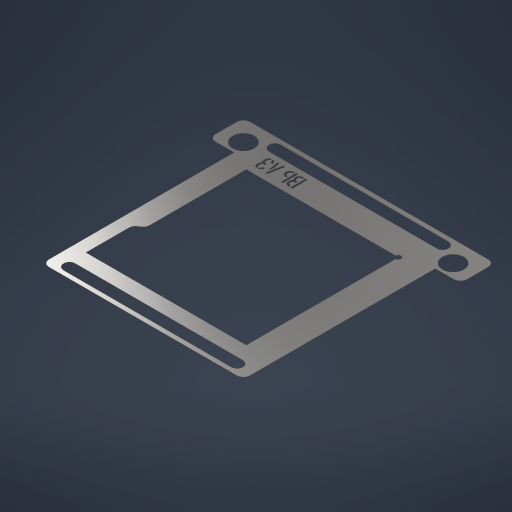
# Autodesk Inventor part: Baseplate Film Stencil - V1
Saved by Autodesk Inventor 2024 (Build 280153000, 153)
## iProperties
Created: 2022-06-23
Part Number: Baseplate Film Stencil - V1
Material: Stainless Steel
Document SubType Name: Modeling
Designer: Caleb
Density: 8 g/cm^3
Appearance: Semi-Polished
Author: Caleb
Autodesk Inventor part; units mm, degrees
ref_plane "YZ Plane" through (0, 0, 0) normal (1, 0, 0) x (0, 1, 0)
ref_plane "XZ Plane" through (0, 0, 0) normal (0, 1, 0) x (-1, 0, 0)
ref_plane "XY Plane" through (0, 0, 0) normal (0, 0, 1) x (1, 0, 0)
sketch "Sketch1" plane through (0, 0, 0) normal (0, 1, 0) x (-1, 0, 0)
  line L0 (-38.1, -34.29) -> (38.1, -34.29)
  line L1 (38.1, -34.29) -> (38.1, 34.29)
  line L2 (38.1, 34.29) -> (-38.1, 34.29)
  line L3 (-38.1, 34.29) -> (-38.1, -34.29)
  line L4 (-38.1, -34.29) -> (38.1, 34.29) construction
  line L5 (38.1, -34.29) -> (-38.1, 34.29) construction
  point P0 (0, 0)
  dimension "d0" = 76.2
  dimension "d1" = 68.58
  constraints: 12 end point, 2 midpoint, 2 parallel, 1 horizontal, 1 perpendicular
  measures "d0" distance of L2.end L1.end
  measures "d1" distance of L1.end L0.end
extrude "Extrusion1" add sketch "Sketch1" along normal blind 0.0508
sketch "Sketch2" plane through (0, 0.0508, 0) normal (0, 1, 0) x (1, 0, 0)
  line L0 (-38.1, -34.29) -> (38.1, -34.29) projected
  line L1 (-46.3971, 0) -> (43.7494, 0)
  line L2 (-38.1, 34.29) -> (-38.1, -34.29) projected
  line L3 (38.1, -34.29) -> (38.1, 34.29) projected
  line L4 (38.1, 23.79) -> (30.48, 23.79)
  line L5 (30.48, 23.79) -> (30.48, -34.29)
  line L6 (30.48, -34.29) -> (38.1, -34.29)
  line L7 (38.1, -34.29) -> (38.1, 23.79)
  line L8 (0, -45.6355) -> (0, 71.8702)
  line L9 (46.3971, 0) -> (-43.7494, 0)
  line L10 (-38.1, -34.29) -> (-38.1, 34.29)
  line L11 (-38.1, 23.79) -> (-30.48, 23.79)
  line L12 (-30.48, 23.79) -> (-30.48, -34.29)
  line L13 (-30.48, -34.29) -> (-38.1, -34.29)
  line L14 (-38.1, -34.29) -> (-38.1, 23.79)
  line L15 (38.1, 34.29) -> (-38.1, 34.29) projected
  point P0 (0, 0)
  point P1 (38.1, -27.305)
  dimension "d14" = 7.62
  dimension "d16" = 10.5
  constraints: 24 end point, 6 symmetric about line, 3 point on line, 2 horizontal, 2 parallel, 1 perpendicular, 1 vertical
  measures "d14" distance of L5.end L6.end
  measures "d16" distance between parallel lines of L15 L4
extrude "Extrusion2" cut sketch "Sketch2" against normal through all contours L2 L1 L12 L0 | L2 L11 L12 L1 | L5 L1 L3 L0 | L5 L4 L3 L1
sketch "Sketch6" plane through (0, 0.0508, 0) normal (0, 1, 0) x (1, 0, 0)
  line L0 (38.1, 34.29) -> (-38.1, 34.29) projected
  line L1 (-38.1, 34.29) -> (-38.1, 23.79) projected
  line L2 (38.1, 23.79) -> (38.1, 34.29) projected
  point P0 (0, 0)
  point P1 (-31.75, 27.94)
  point P2 (31.75, 27.94)
  point P3 (36.1, 34.29)
  point P4 (-36.1, 34.29)
  point P5 (-38.1, 32.29)
  point P6 (-38.1, 25.29)
  point P7 (38.1, 25.29)
  point P8 (38.1, 32.29)
  point P9 (38.1, 28.79)
  dimension "d41" = 6.35
  dimension "d42" = 6.35
  dimension "d43" = 6.35
  constraints: 1 horizontal alignment, 1 point on line
  measures "d41" distance from line of L0 point (-31.75, 27.94)
  measures "d42" distance from line of L1 point (-31.75, 27.94)
  measures "d43" horizontal distance of point (38.1, 28.79) point (31.75, 27.94)
hole "Hole1" at (-31.75, 0.0508, -27.94) at (31.75, 0.0508, -27.94) direction (0, -1, 0) diameter 6.477 end through all
sketch "Sketch3" plane through (0, 0.0508, 0) normal (0, 1, 0) x (1, 0, 0)
  line L0 (25.4, -31.115) -> (-25.4, -31.115) construction
  line L1 (25.4, -29.365) -> (-25.4, -29.365)
  line L2 (-25.4, -32.865) -> (25.4, -32.865)
  arc A0 (25.4, -32.865) -> (25.4, -29.365) centre (25.4, -31.115) ccw
  arc A1 (-25.4, -29.365) -> (-25.4, -32.865) centre (-25.4, -31.115) ccw
  line L3 (25.4, 31.115) -> (-25.4, 31.115) construction
  line L4 (25.4, 32.865) -> (-25.4, 32.865)
  line L5 (-25.4, 29.365) -> (25.4, 29.365)
  arc A2 (25.4, 29.365) -> (25.4, 32.865) centre (25.4, 31.115) ccw
  arc A3 (-25.4, 32.865) -> (-25.4, 29.365) centre (-25.4, 31.115) ccw
  line L6 (38.1, 34.29) -> (-38.1, 34.29) projected
  line L7 (-38.1, -34.29) -> (38.1, -34.29) projected
  point P0 (0, 0)
  point P1 (0, -31.115)
  point P2 (0, 31.115)
  dimension "d17" = 3.5
  dimension "d18" = 3.5
  dimension "d19" = 50.8
  dimension "d20" = 50.8
  dimension "d21" = 3.175
  dimension "d22" = 3.175
  constraints: 16 end point, 8 point on circle, 8 tangent, 4 centre point, 3 parallel, 2 midpoint, 2 vertical alignment, 1 horizontal
  measures "d17" distance between parallel lines of L2 L1
  measures "d18" distance between parallel lines of L4 L5
  measures "d19" distance of L0.end L0.start
  measures "d20" distance of L3.end L3.start
  measures "d21" distance from line of L6 point (0, 31.115)
  measures "d22" distance from line of L7 point (0, -31.115)
extrude "Extrusion3" cut sketch "Sketch3" against normal through all
sketch "Sketch4" plane through (0, 0.0508, 0) normal (0, 1, 0) x (1, 0, 0)
  line L0 (-24.105, -24.825) -> (21.895, -24.825)
  line L1 (21.895, -24.825) -> (21.895, 21.175)
  line L2 (21.895, 21.175) -> (-24.105, 21.175)
  line L3 (-24.105, 21.175) -> (-24.105, -24.825)
  line L4 (38.1, 34.29) -> (-38.1, 34.29) projected
  line L5 (38.1, 23.79) -> (38.1, 34.29) projected
  circle A0 centre (21.895, 21.175) radius 0.7938
  circle A1 centre (31.75, 27.94) radius 3.2385 projected
  point P0 (0, 0)
  point P1 (21.895, 20.3813)
  point P2 (21.1012, 21.175)
  point P3 (29.845, 22.225)
  dimension "d29" = 1.5875
  dimension "d34" = 46
  dimension "d35" = 46
  dimension "d51" = 1.905
  dimension "d52" = 5.715
  dimension "d53" = 7.95
  dimension "d54" = 1.05
  constraints: 8 end point, 2 parallel, 1 centre point, 1 coincident, 1 horizontal, 1 perpendicular
  measures "d29" diameter of A0
  measures "d34" distance of L0.start L0.end
  measures "d35" distance of L2.end L0.start
  measures "d51" horizontal distance of point (29.845, 22.225) A1.centre
  measures "d52" vertical distance of point (29.845, 22.225) A1.centre
  measures "d53" distance from line of L1 point (29.845, 22.225)
  measures "d54" distance from line of L2 point (29.845, 22.225)
extrude "Extrusion4" cut sketch "Sketch4" against normal through all contours L3 L2 A0 L1 L0 | A0 L2 L1 | L1 L2 A0
sketch "Sketch5" plane through (0, 0.0508, 0) normal (0, 1, 0) x (1, 0, 0)
  line L0 (-24.105, -24.825) -> (-24.105, 21.175) projected
  line L1 (-24.105, -24.825) -> (-26.605, -24.825)
  line L2 (-26.605, -24.825) -> (-26.605, -9.825)
  line L3 (-26.605, -9.825) -> (-24.105, -9.825)
  line L4 (-24.105, -9.825) -> (-24.105, -24.825)
  point P0 (0, 0)
  point P1 (-24.105, -9.825)
  dimension "d36" = 15
  dimension "d37" = 2.5
  constraints: 8 end point, 2 parallel, 1 horizontal, 1 perpendicular
  measures "d36" distance of L1.end L2.end
  measures "d37" distance of L2.end L3.end
extrude "Extrusion5" cut sketch "Sketch5" against normal through all
fillet "Fillet2" radius 2 8 edges at (30.48, 0.0254, 34.29) (-30.48, 0.0254, 34.29) (-38.1, 0.0254, -23.79) (-38.1, 0.0254, -34.29) (38.1, 0.0254, -34.29) (38.1, 0.0254, -23.79) (-24.105, 0.0254, 9.825) (-26.605, 0.0254, 9.825)
sketch "Sketch8" plane through (0, 0, 0) normal (0, -1, 0) x (1, 0, 0)
  line L0 (-11.9362, -27.7477) -> (-25.3264, -27.7477) construction
  line L1 (-25.3264, -27.7477) -> (-25.3264, -23.0961) construction
  line L2 (-25.3264, -23.0961) -> (-11.9362, -23.0961) construction
  line L3 (-11.9362, -23.0961) -> (-11.9362, -27.7477) construction
  spline S0 degree 2 poles (-13.4121, -27.2933) (-13.6942, -27.287) (-14.0545, -26.9799) (-14.0608, -26.748) knots 0 0 0 1 2 2 2
  line L4 (-14.0608, -26.748) -> (-14.0608, -26.2717)
  spline S1 degree 2 poles (-14.0608, -26.2717) (-14.0545, -26.043) (-13.6816, -25.739) (-13.3996, -25.7327) knots 0 0 0 1 2 2 2
  line L5 (-13.3996, -25.7327) -> (-13.221, -25.7327)
  line L6 (-13.221, -25.7327) -> (-13.221, -25.2313)
  line L7 (-13.221, -25.2313) -> (-13.3996, -25.2313)
  spline S2 degree 2 poles (-13.3996, -25.2313) (-13.6816, -25.2251) (-14.0545, -24.918) (-14.0608, -24.6861) knots 0 0 0 1 2 2 2
  line L8 (-14.0608, -24.6861) -> (-14.0608, -24.2129)
  spline S3 degree 2 poles (-14.0608, -24.2129) (-14.0545, -23.9873) (-13.6816, -23.7146) (-13.3996, -23.7115) knots 0 0 0 1 2 2 2
  line L9 (-13.3996, -23.7115) -> (-13.221, -23.7115)
  line L10 (-13.221, -23.7115) -> (-13.221, -23.2226)
  line L11 (-13.221, -23.2226) -> (-13.3996, -23.2226)
  spline S4 degree 2 poles (-13.3996, -23.2226) (-13.6879, -23.2226) (-14.2457, -23.4577) (-14.6123, -23.9026) (-14.6186, -24.2191) knots 0 0 0 1 2 3 3 3
  line L12 (-14.6186, -24.2191) -> (-14.6186, -24.7174)
  spline S5 degree 2 poles (-14.6186, -24.7174) (-14.6155, -24.9462) (-14.3898, -25.341) (-14.1893, -25.482) knots 0 0 0 1 2 2 2
  spline S6 degree 2 poles (-14.1893, -25.482) (-14.3898, -25.6199) (-14.6155, -26.0116) (-14.6186, -26.2404) knots 0 0 0 1 2 2 2
  line L13 (-14.6186, -26.2404) -> (-14.6186, -26.7418)
  spline S7 degree 2 poles (-14.6186, -26.7418) (-14.6123, -27.0551) (-14.2426, -27.5001) (-13.6848, -27.7414) (-13.3996, -27.7414) knots 0 0 0 1 2 3 3 3
  line L14 (-13.3996, -27.7414) -> (-13.221, -27.7414)
  line L15 (-13.221, -27.7414) -> (-13.221, -27.2933)
  line L16 (-13.221, -27.2933) -> (-13.4121, -27.2933)
  line L17 (-12.4689, -23.2226) -> (-12.7008, -23.2226)
  line L18 (-12.7008, -23.2226) -> (-12.7008, -27.7414)
  line L19 (-12.7008, -27.7414) -> (-12.4689, -27.7414)
  spline S8 degree 2 poles (-12.4689, -27.7414) (-12.3341, -27.7414) (-12.1806, -27.6443) (-12.1806, -27.5315) knots 0 0 0 1 2 2 2
  line L20 (-12.1806, -27.5315) -> (-12.1806, -23.4357)
  spline S9 degree 2 poles (-12.1806, -23.4357) (-12.1806, -23.3166) (-12.3341, -23.2226) (-12.4689, -23.2226) knots 0 0 0 1 2 2 2
  line L21 (-15.2736, -23.2226) -> (-15.4114, -23.2226)
  spline S10 degree 2 poles (-15.4114, -23.2226) (-15.4898, -23.2258) (-15.5995, -23.3198) (-15.6026, -23.3887) knots 0 0 0 1 2 2 2
  line L22 (-15.6026, -23.3887) -> (-15.6026, -27.7414)
  line L23 (-15.6026, -27.7414) -> (-15.2736, -27.7414)
  spline S11 degree 2 poles (-15.2736, -27.7414) (-15.1952, -27.7383) (-15.0855, -27.6411) (-15.0824, -27.5691) knots 0 0 0 1 2 2 2
  line L24 (-15.0824, -27.5691) -> (-15.0824, -23.3887)
  spline S12 degree 2 poles (-15.0824, -23.3887) (-15.0855, -23.3198) (-15.1952, -23.2258) (-15.2736, -23.2226) knots 0 0 0 1 2 2 2
  line L25 (-16.1165, -25.6732) -> (-16.1165, -25.2313)
  line L26 (-16.1165, -25.2313) -> (-16.245, -25.2313)
  spline S13 degree 2 poles (-16.245, -25.2313) (-16.5176, -25.2313) (-17.0347, -25.457) (-17.3825, -25.8737) (-17.4045, -26.1683) knots 0 0 0 1 2 3 3 3
  spline S14 degree 2 poles (-17.4045, -26.1683) (-17.4139, -26.4754) (-17.4045, -26.7856) knots 0 0 0 1 1 1
  spline S15 degree 2 poles (-17.4045, -26.7856) (-17.3888, -27.0802) (-17.041, -27.5064) (-16.5176, -27.7383) (-16.245, -27.7414) knots 0 0 0 1 2 3 3 3
  line L27 (-16.245, -27.7414) -> (-16.1165, -27.7414)
  line L28 (-16.1165, -27.7414) -> (-16.1165, -27.2933)
  line L29 (-16.1165, -27.2933) -> (-16.2575, -27.2933)
  spline S16 degree 2 poles (-16.2575, -27.2933) (-16.5239, -27.287) (-16.8717, -26.9799) (-16.878, -26.748) knots 0 0 0 1 2 2 2
  spline S17 degree 2 poles (-16.878, -26.748) (-16.8905, -26.6164) (-16.8811, -26.3532) (-16.878, -26.2184) knots 0 0 0 1 2 2 2
  spline S18 degree 2 poles (-16.878, -26.2184) (-16.8717, -25.9928) (-16.5239, -25.6795) (-16.2575, -25.6732) knots 0 0 0 1 2 2 2
  line L30 (-16.2575, -25.6732) -> (-16.1165, -25.6732)
  line L31 (-18.9964, -27.6443) -> (-19.83, -23.326)
  spline S19 degree 2 poles (-19.83, -23.326) (-19.8519, -23.2508) (-19.9208, -23.2195) (-19.971, -23.2226) knots 0 0 0 1 2 2 2
  line L32 (-19.971, -23.2226) -> (-20.2561, -23.2226)
  spline S20 degree 2 poles (-20.2561, -23.2226) (-20.2875, -23.2226) (-20.3314, -23.2289) (-20.3502, -23.2414) knots 0 0 0 1 2 2 2
  line L33 (-20.3502, -23.2414) -> (-19.8362, -25.9646)
  line L34 (-19.8362, -25.9646) -> (-19.5103, -27.6568)
  spline S21 degree 2 poles (-19.5103, -27.6568) (-19.5009, -27.707) (-19.4602, -27.7383) (-19.4132, -27.7414) knots 0 0 0 1 2 2 2
  line L35 (-19.4132, -27.7414) -> (-19.0935, -27.7414)
  spline S22 degree 2 poles (-19.0935, -27.7414) (-19.0403, -27.7414) (-18.987, -27.7007) (-18.9964, -27.6443) knots 0 0 0 1 2 2 2
  line L36 (-20.6197, -24.545) -> (-21.2182, -27.6317)
  spline S23 degree 2 poles (-21.2182, -27.6317) (-21.2276, -27.6944) (-21.19, -27.7414) (-21.1461, -27.7414) knots 0 0 0 1 2 2 2
  line L37 (-21.1461, -27.7414) -> (-20.8265, -27.7414)
  spline S24 degree 2 poles (-20.8265, -27.7414) (-20.7826, -27.7414) (-20.7199, -27.7007) (-20.7043, -27.638) knots 0 0 0 1 2 2 2
  line L38 (-20.7043, -27.638) -> (-20.369, -25.8988)
  line L39 (-20.369, -25.8988) -> (-20.6197, -24.545)
  spline S25 degree 2 poles (-22.8007, -25.2501) (-22.9574, -25.2501) (-23.2363, -25.1154) (-23.4149, -24.871) (-23.4181, -24.7111) knots 0 0 0 1 2 3 3 3
  line L40 (-23.4181, -24.7111) -> (-23.4181, -24.1815)
  spline S26 degree 2 poles (-23.4181, -24.1815) (-23.4149, -24.0186) (-23.2206, -23.7585) (-23.0577, -23.6927) knots 0 0 0 1 2 2 2
  line L41 (-23.0577, -23.6927) -> (-23.0577, -23.2226)
  spline S27 degree 2 poles (-23.0577, -23.2226) (-23.3146, -23.2759) (-23.7064, -23.5611) (-23.9288, -23.9653) (-23.932, -24.1941) knots 0 0 0 1 2 3 3 3
  line L42 (-23.932, -24.1941) -> (-23.932, -24.6955)
  spline S28 degree 2 poles (-23.932, -24.6955) (-23.9288, -24.9305) (-23.7001, -25.341) (-23.4964, -25.4883) knots 0 0 0 1 2 2 2
  spline S29 degree 2 poles (-23.4964, -25.4883) (-23.7001, -25.6324) (-23.9288, -26.043) (-23.932, -26.2717) knots 0 0 0 1 2 2 2
  line L43 (-23.932, -26.2717) -> (-23.932, -26.7794)
  spline S30 degree 2 poles (-23.932, -26.7794) (-23.9288, -27.0081) (-23.7001, -27.4061) (-23.3084, -27.6913) (-23.0577, -27.7477) knots 0 0 0 1 2 3 3 3
  line L44 (-23.0577, -27.7477) -> (-23.0577, -27.2808)
  spline S31 degree 2 poles (-23.0577, -27.2808) (-23.2206, -27.2087) (-23.4149, -26.9517) (-23.4181, -26.7856) knots 0 0 0 1 2 2 2
  line L45 (-23.4181, -26.7856) -> (-23.4181, -26.2592)
  spline S32 degree 2 poles (-23.4181, -26.2592) (-23.4149, -26.0962) (-23.2332, -25.8549) (-22.9543, -25.7202) (-22.8007, -25.7202) knots 0 0 0 1 2 3 3 3
  spline S33 degree 2 poles (-22.8007, -25.7202) (-22.644, -25.7202) (-22.5406, -25.6669) (-22.5469, -25.6042) knots 0 0 0 1 2 2 2
  line L46 (-22.5469, -25.6042) -> (-22.5469, -25.4883)
  spline S34 degree 2 poles (-22.5469, -25.4883) (-22.5437, -25.4131) (-22.5469, -25.3065) (-22.6534, -25.2501) (-22.8007, -25.2501) knots 0 0 0 1 2 3 3 3
  line L47 (-21.6726, -26.8546) -> (-21.6726, -26.7794)
  spline S35 degree 2 poles (-21.6726, -26.7794) (-21.6694, -26.6728) (-21.729, -26.6133) (-21.8261, -26.6196) knots 0 0 0 1 2 2 2
  spline S36 degree 2 poles (-21.8261, -26.6196) (-21.8512, -26.6196) (-21.9013, -26.6196) (-21.9295, -26.6196) knots 0 0 0 1 2 2 2
  spline S37 degree 2 poles (-21.9295, -26.6196) (-21.9765, -26.6196) (-22.0079, -26.6196) knots 0 0 0 1 1 1
  spline S38 degree 2 poles (-22.0079, -26.6196) (-22.127, -26.6133) (-22.1928, -26.6728) (-22.1928, -26.7856) knots 0 0 0 1 2 2 2
  spline S39 degree 2 poles (-22.1928, -26.7856) (-22.1959, -26.9517) (-22.3839, -27.2087) (-22.5469, -27.2808) knots 0 0 0 1 2 2 2
  line L48 (-22.5469, -27.2808) -> (-22.5469, -27.7477)
  spline S40 degree 2 poles (-22.5469, -27.7477) (-22.1834, -27.6631) (-21.707, -27.1805) (-21.6726, -26.8546) knots 0 0 0 1 2 2 2
  spline S41 degree 2 poles (-22.5531, -23.2226) (-22.5469, -23.232) (-22.5469, -23.2508) (-22.5469, -23.2602) knots 0 0 0 1 2 2 2
  line L49 (-22.5469, -23.2602) -> (-22.5469, -23.6989)
  spline S42 degree 2 poles (-22.5469, -23.6989) (-22.3839, -23.7616) (-22.1959, -24.0186) (-22.1928, -24.1847) knots 0 0 0 1 2 2 2
  spline S43 degree 2 poles (-22.1928, -24.1847) (-22.1959, -24.2912) (-22.1489, -24.357) (-22.0706, -24.3508) knots 0 0 0 1 2 2 2
  spline S44 degree 2 poles (-22.0706, -24.3508) (-22.0236, -24.3508) (-21.9358, -24.3508) knots 0 0 0 1 1 1
  spline S45 degree 2 poles (-21.9358, -24.3508) (-21.8982, -24.3508) (-21.8355, -24.3508) (-21.8073, -24.3508) knots 0 0 0 1 2 2 2
  spline S46 degree 2 poles (-21.8073, -24.3508) (-21.7227, -24.357) (-21.6694, -24.3006) (-21.6726, -24.1972) knots 0 0 0 1 2 2 2
  spline S47 degree 2 poles (-21.6726, -24.1972) (-21.6757, -23.9684) (-21.8982, -23.5673) (-22.2931, -23.279) (-22.5531, -23.2226) knots 0 0 0 1 2 3 3 3
  point P0 (0, 0)
  dimension "d0" = 76.2
  dimension "d1" = 68.58
  constraints: 2 other
emboss "Emboss2" sketch "Sketch8" operation cut depth 1 direction (0, 1, 0)
equation "\"d42\" = d41"
equation "\"d43\" = d42"
equation "\"d18\" = d17"
equation "\"d20\" = d19"
body "Solid1"
